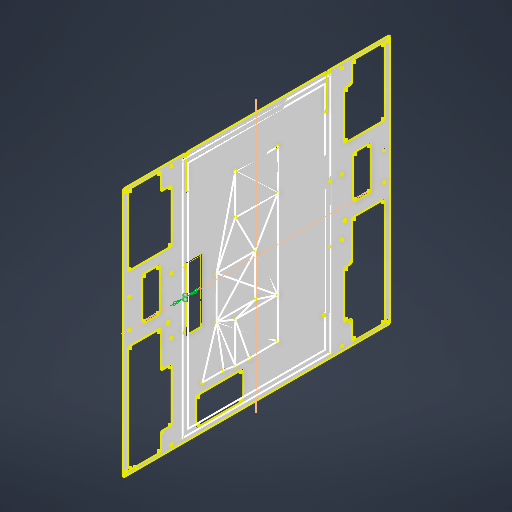
# Autodesk Inventor part: дно 25-26
Saved by Autodesk Inventor 2026.2 (Build 302298000, 298)
## iProperties
Created: 2025-09-06
Part Number: дно 25-26
Material: Типовые
Document SubType Name: Modeling
Designer: Trene
Density: 1 g/cm^3
Appearance: По умолчанию
Author: Trene
Autodesk Inventor part; units mm, degrees
(part 1 of 4)
ref_plane "YZ Plane" through (0, 0, 0) normal (1, 0, 0) x (0, 1, 0)
ref_plane "XZ Plane" through (0, 0, 0) normal (0, 1, 0) x (-1, 0, 0)
ref_plane "XY Plane" through (0, 0, 0) normal (0, 0, 1) x (1, 0, 0)
sketch "Эскиз1" plane through (0, 0, 0) normal (1, 0, 0) x (0, 1, 0)
  line L0 (0, 0) -> (370, 0)
  line L1 (370, 0) -> (370, -370)
  line L2 (370, -370) -> (0, -370)
  line L3 (0, -370) -> (0, 0)
  dimension "d0" = 370
  dimension "d1" = 370
  constraints: 8 end point, 2 parallel, 1 horizontal, 1 perpendicular
  measures "d0" distance of L1.end L2.end
  measures "d1" distance of L0.end L1.end
extrude "Выдавливание1" add sketch "Эскиз1" along normal blind 1.5
sketch "Эскиз3" plane through (1.5, 0, 0) normal (1, 0, 0) x (0, 0, -1)
  line L0 (0, 0) -> (370, 0) projected
  line L1 (8, 0) -> (50, 0)
  line L2 (50, 0) -> (50, 100)
  line L3 (50, 100) -> (8, 100)
  line L4 (8, 100) -> (8, 0)
  line L5 (0, 370) -> (0, 0) projected
  line L6 (370, 370) -> (0, 370) projected
  line L7 (185, 370) -> (185, 0)
  line L8 (0, 185) -> (370, 185)
  line L9 (370, 0) -> (370, 370) projected
  line L10 (362, 0) -> (320, 0)
  line L11 (320, 0) -> (320, 100)
  line L12 (320, 100) -> (362, 100)
  line L13 (362, 100) -> (362, 0)
  line L14 (8, 370) -> (50, 370)
  line L15 (50, 370) -> (50, 270)
  line L16 (50, 270) -> (8, 270)
  line L17 (8, 270) -> (8, 370)
  line L18 (362, 370) -> (320, 370)
  line L19 (320, 370) -> (320, 270)
  line L20 (320, 270) -> (362, 270)
  line L21 (362, 270) -> (362, 370)
  point P0 (362, 370)
  point P1 (8, 370)
  dimension "d9" = 42
  dimension "d10" = 100
  dimension "d13" = 8
  constraints: 36 end point, 12 symmetric about line, 4 midpoint, 2 parallel, 1 horizontal, 1 perpendicular, 1 point on line
  measures "d9" distance of L3.end L2.end
  measures "d10" distance of L2.end L1.end
  measures "d13" distance between parallel lines of L5 L4
extrude "Выдавливание3" cut sketch "Эскиз3" against normal blind 10 contours L4 L3 L2 L0 | L6 L15 L16 L17 | L11 L12 L13 L0 | L6 L21 L20 L19
sketch "Эскиз4" plane through (1.5, 0, 0) normal (1, 0, 0) x (0, 0, -1)
  line L0 (50, 0) -> (320, 0) projected
  line L1 (185, 0) -> (185, 257.6138)
  line L2 (0, 370) -> (0, 0) projected
  line L3 (0, 185) -> (403.9864, 185)
  line L4 (120, 370.5966) -> (250, 370.5966)
  line L5 (250, 370.5966) -> (250, 320.5966)
  line L6 (250, 320.5966) -> (120, 320.5966)
  line L7 (120, 320.5966) -> (120, 370.5966)
  line L8 (120, 370.5966) -> (250, 320.5966) construction
  line L9 (250, 370.5966) -> (120, 320.5966) construction
  point P0 (185, 370)
  point P1 (185, 305.5966)
  dimension "d62" = 50
  dimension "d63" = 130
  constraints: 12 end point, 2 midpoint, 1 horizontal, 1 symmetric about line, 1 vertical, 6 other
  measures "d62" distance between parallel lines of L4 L6
  measures "d63" distance between parallel lines of L7 L5
extrude "Выдавливание4" cut sketch "Эскиз4" against normal blind 10
sketch "Эскиз5" plane through (1.5, 0, 0) normal (1, 0, 0) x (0, 0, -1)
  line L0 (320, 370) -> (250, 370) projected
  line L1 (50, 0) -> (320, 0) projected
  line L2 (185, 0) -> (185, 405.4433)
  line L3 (50, 100) -> (50, 0) projected
  line L4 (320, 100) -> (362, 100) projected
  line L5 (320, 100) -> (362, 100)
  line L6 (362, 100) -> (362, 103)
  line L7 (362, 103) -> (320, 103)
  line L8 (320, 103) -> (320, 100)
  line L9 (50, 100) -> (8, 100)
  line L10 (50, 100) -> (8, 100)
  line L11 (8, 100) -> (8, 103)
  line L12 (8, 103) -> (50, 103)
  line L13 (50, 103) -> (50, 100)
  line L14 (0, 370) -> (0, 0) projected
  line L15 (0, 185) -> (370, 185)
  line L16 (370, 0) -> (370, 370) projected
  line L17 (50, 270) -> (50, 370)
  line L18 (320, 270) -> (362, 270)
  line L19 (320, 270) -> (362, 270)
  line L20 (362, 270) -> (362, 267)
  line L21 (362, 267) -> (320, 267)
  line L22 (320, 267) -> (320, 270)
  line L23 (50, 267) -> (50, 270)
  line L24 (8, 267) -> (50, 267)
  line L25 (50, 270) -> (8, 270)
  line L26 (50, 270) -> (8, 270)
  line L27 (8, 270) -> (8, 267)
  line L28 (320, 0) -> (320, 100) projected
  line L29 (362, 103) -> (320, 103)
  line L30 (320, 103) -> (320, 140)
  line L31 (320, 140) -> (362, 140)
  line L32 (362, 140) -> (362, 103)
  line L33 (8, 103) -> (50, 103)
  line L34 (50, 103) -> (50, 140)
  line L35 (50, 140) -> (8, 140)
  line L36 (8, 140) -> (8, 103)
  point P0 (250, 0)
  point P1 (185, -35.4433)
  dimension "d36" = 42
  dimension "d37" = 3
  constraints: 60 end point, 21 symmetric about line, 4 parallel, 3 midpoint, 2 horizontal, 2 perpendicular, 1 vertical
  measures "d36" distance of L7.end L6.end
  measures "d37" distance of L6.end L5.end
extrude "Выдавливание5" cut sketch "Эскиз5" against normal blind 10 contours L30 L31 L32 L7 | L12 L36 L35 L34
sketch "Эскиз6" plane through (1.5, 0, 0) normal (1, 0, 0) x (0, 0, -1)
  line L0 (320, 370) -> (250, 370) projected
  line L1 (299, 370) -> (259, 370)
  line L2 (259, 370) -> (259, 355)
  line L3 (259, 355) -> (299, 355)
  line L4 (299, 355) -> (299, 370)
  line L5 (250, 320.5966) -> (120, 320.5966) projected
  line L6 (185, 320.5966) -> (185, 152.8583)
  line L7 (71, 370) -> (111, 370)
  line L8 (111, 370) -> (111, 355)
  line L9 (111, 355) -> (71, 355)
  line L10 (71, 355) -> (71, 370)
  line L11 (95.25, 0) -> (95.25, 55) projected
  line L12 (95.25, 0) -> (163.25, 0)
  line L13 (163.25, 0) -> (163.25, 15)
  line L14 (163.25, 15) -> (95.25, 15)
  line L15 (95.25, 15) -> (95.25, 0)
  line L16 (8, 0) -> (50, 0)
  line L17 (50, 0) -> (50, 3)
  line L18 (50, 3) -> (8, 3)
  line L19 (8, 3) -> (8, 0)
  line L20 (362, 0) -> (320, 0)
  line L21 (320, 0) -> (320, 3)
  line L22 (320, 3) -> (362, 3)
  line L23 (362, 3) -> (362, 0)
  line L24 (370, 0) -> (370, 370) projected
  line L25 (370, 0) -> (0, 0)
  line L26 (0, 0) -> (0, -2)
  line L27 (0, -2) -> (370, -2)
  line L28 (370, -2) -> (370, 0)
  line L29 (0, 370) -> (0, 0) projected
  line L30 (0, 185) -> (370, 185)
  line L31 (370, 370) -> (0, 370)
  line L32 (0, 370) -> (0, 372)
  line L33 (0, 372) -> (370, 372)
  line L34 (370, 372) -> (370, 370)
  line L35 (50, 370) -> (50, 367)
  line L36 (50, 367) -> (8, 367)
  line L37 (8, 367) -> (8, 370)
  line L38 (320, 370) -> (320, 367)
  line L39 (320, 367) -> (362, 367)
  line L40 (362, 367) -> (362, 370)
  point P0 (362, 370)
  dimension "d28" = 40
  dimension "d29" = 15
  dimension "d32" = 68
  dimension "d33" = 15
  dimension "d34" = 42
  dimension "d35" = 3
  dimension "d38" = 370
  dimension "d39" = 2
  constraints: 72 end point, 18 symmetric about line, 8 parallel, 4 horizontal, 4 perpendicular, 3 midpoint, 1 vertical
  measures "d28" distance of L3.end L2.end
  measures "d29" distance of L2.end L1.end
  measures "d32" distance of L14.end L13.end
  measures "d33" distance of L13.end L12.end
  measures "d34" distance of L18.end L17.end
  measures "d35" distance of L17.end L16.end
  measures "d38" distance of L27.end L26.end
  measures "d39" distance of L26.end L25.end
extrude "Выдавливание6" add sketch "Эскиз6" against normal up to surface (1.5 mm away) contours L0 L31 L7 L32 L33 L34 | L31 L40 L39 L38 | L4 L3 L2 L0 | L8 L9 L10 L7 | L28 L27 L26 L25 L16 L12 L20 | L20 L21 L22 L23 | L35 L36 L37 L31 | L12 L11 L14 L13 | L19 L18 L17 L16
sketch "Эскиз7" plane through (0, 0, 0) normal (-1, 0, 0) x (0, 0, 1)
  line L0 (0, -2) -> (0, 372) projected
  line L1 (0, 372) -> (-370, 372) projected
  line L2 (-370, -2) -> (-370, 372) projected
  line L3 (-370, -2) -> (0, -2) projected
  line L4 (-362, 3) -> (-362, 100) projected
  line L5 (-320, 100) -> (-320, 3) projected
  line L6 (-320, 3) -> (-362, 3) projected
  line L7 (-320, 367) -> (-320, 270) projected
  line L8 (-362, 270) -> (-362, 367) projected
  line L9 (-362, 367) -> (-320, 367) projected
  line L10 (-250, 370) -> (-120, 370) projected
  line L11 (-120, 370) -> (-120, 320.5966) projected
  line L12 (-120, 320.5966) -> (-250, 320.5966) projected
  line L13 (-250, 320.5966) -> (-250, 370) projected
  line L14 (-8, 3) -> (-50, 3) projected
  line L15 (-50, 3) -> (-50, 100) projected
  line L16 (-8, 100) -> (-8, 3) projected
  line L17 (-50, 367) -> (-8, 367) projected
  line L18 (-8, 367) -> (-8, 270) projected
  line L19 (-50, 270) -> (-50, 367) projected
  line L20 (0, 15) -> (-370, 15)
  line L21 (-362, 100) -> (-320, 100) projected
  line L22 (-320, 270) -> (-362, 270) projected
  line L23 (-50, 100) -> (-8, 100) projected
  line L24 (-8, 270) -> (-50, 270) projected
  point P0 (0, 0)
  point P1 (-8, 15)
  point P2 (-50, 15)
  point P3 (-320, 15)
  point P4 (-362, 15)
  constraints: 2 end point, 2 point on line, 1 perpendicular
extrude "Выдавливание7" cut sketch "Эскиз7" against normal blind 10 contours L3 L2 L20 L4 L6 L5 L15 L14 L16 L0 | L20 L15 L23 L16 | L16 L14 L15 L20 | L20 L5 L6 L4
sketch "Эскиз8" plane through (1.5, 0, 0) normal (1, 0, 0) x (0, 0, -1)
  line L0 (8, 103) -> (8, 140) projected
  line L1 (8, 140) -> (50, 140) projected
  line L2 (50, 140) -> (50, 103) projected
  line L3 (50, 103) -> (8, 103) projected
  line L4 (320, 103) -> (320, 140) projected
  line L5 (320, 140) -> (362, 140) projected
  line L6 (362, 140) -> (362, 103) projected
  line L7 (362, 103) -> (320, 103) projected
  line L8 (8, 367) -> (50, 367) projected
  line L9 (50, 367) -> (50, 270) projected
  line L10 (50, 270) -> (8, 270) projected
  line L11 (8, 270) -> (8, 367) projected
  line L12 (362, 15) -> (370, 15) projected
  line L13 (370, 15) -> (370, 372) projected
  line L14 (370, 372) -> (0, 372) projected
  line L15 (0, 372) -> (0, 15) projected
  line L16 (0, 15) -> (8, 15) projected
  line L17 (8, 15) -> (8, 100) projected
  line L18 (8, 100) -> (50, 100) projected
  line L19 (50, 100) -> (50, 15) projected
  line L20 (50, 15) -> (320, 15) projected
  line L21 (320, 15) -> (320, 100) projected
  line L22 (320, 100) -> (362, 100) projected
  line L23 (362, 100) -> (362, 15) projected
  line L24 (320, 367) -> (362, 367) projected
  line L25 (362, 367) -> (362, 270) projected
  line L26 (362, 270) -> (320, 270) projected
  line L27 (320, 270) -> (320, 367) projected
  line L28 (250, 370) -> (250, 320.5966) projected
  line L29 (250, 320.5966) -> (120, 320.5966) projected
  line L30 (120, 320.5966) -> (120, 370) projected
  line L31 (120, 370) -> (250, 370) projected
  line L32 (362, 100) -> (362, 103)
  line L33 (320, 100) -> (320, 103)
  line L34 (50, 100) -> (50, 103)
  line L35 (8, 100) -> (8, 103)
  line L36 (185, 15) -> (113, 15)
  line L37 (113, 15) -> (113, 60)
  line L38 (113, 60) -> (185, 60)
  line L39 (185, 60) -> (185, 15)
  point P0 (0, 0)
  point P1 (113, 15)
  dimension "d54" = 72
  dimension "d55" = 45
  dimension "d58" = 185
  constraints: 16 end point, 5 parallel, 1 horizontal, 1 midpoint, 1 perpendicular, 1 vertical
  measures "d54" distance of L37.end L38.end
  measures "d55" distance of L36.end L37.end
  measures "d58" distance between parallel lines of L15 L39
extrude "Выдавливание8" cut sketch "Эскиз8" against normal blind 10 contours L3 L34 L18 L35 | L37 L38 L39 L20 | L33 L7 L32 L22
ref_plane "РабПлоскость1" through (1.5, 185, 0) normal (0, 1, 0) x (1, 0, 0)
sketch "Эскиз9" plane through (1.5, 0, 0) normal (1, 0, 0) x (0, 0, -1)
  line L0 (50, 140) -> (50, 15) projected
  line L1 (50, 15) -> (113, 15) projected
  line L2 (113, 15) -> (113, 60) projected
  line L3 (113, 60) -> (185, 60) projected
  line L4 (185, 60) -> (185, 15) projected
  line L5 (185, 15) -> (320, 15) projected
  line L6 (320, 15) -> (320, 140) projected
  line L7 (320, 140) -> (362, 140) projected
  line L8 (362, 140) -> (362, 15) projected
  line L9 (362, 15) -> (370, 15) projected
  line L10 (370, 15) -> (370, 372) projected
  line L11 (370, 372) -> (0, 372) projected
  line L12 (0, 372) -> (0, 15) projected
  line L13 (0, 15) -> (8, 15) projected
  line L14 (8, 15) -> (8, 140) projected
  line L15 (8, 140) -> (50, 140) projected
  line L16 (8, 367) -> (50, 367) projected
  line L17 (50, 367) -> (50, 270) projected
  line L18 (50, 270) -> (8, 270) projected
  line L19 (8, 270) -> (8, 367) projected
  line L20 (320, 367) -> (362, 367) projected
  line L21 (362, 367) -> (362, 270) projected
  line L22 (362, 270) -> (320, 270) projected
  line L23 (320, 270) -> (320, 367) projected
  line L24 (250, 370) -> (250, 320.5966) projected
  line L25 (250, 320.5966) -> (120, 320.5966) projected
  line L26 (120, 320.5966) -> (120, 370) projected
  line L27 (120, 370) -> (250, 370) projected
  line L28 (-74, 185) -> (444, 185) projected
  line L29 (8, 3) -> (50, 3)
  line L30 (50, 3) -> (50, 100)
  line L31 (50, 100) -> (8, 100)
  line L32 (8, 100) -> (8, 3)
  line L33 (320, 3) -> (362, 3)
  line L34 (362, 3) -> (362, 100)
  line L35 (362, 100) -> (320, 100)
  line L36 (320, 100) -> (320, 3)
  line L37 (370, -2) -> (0, -2)
  line L38 (370, -2) -> (370, 15)
  line L39 (0, -2) -> (0, 15)
  line L40 (185, 15) -> (113, 15)
  point P0 (0, 0)
  point P1 (50, 15)
  point P2 (8, 15)
  point P3 (362, 15)
  point P4 (320, 15)
  constraints: 24 end point, 10 symmetric about line, 1 collinear, 1 parallel, 1 vertical
extrude "Выдавливание9" add sketch "Эскиз9" against normal up to surface (1.5 mm away) contours L1 L40 L5 L36 L33 L34 L9 L38 L37 L39 L13 L32 L29 L30
sketch "Эскиз10" plane through (1.5, 0, 0) normal (1, 0, 0) x (0, 0, -1)
  point P0 (0, 0)
sketch "Эскиз11" plane through (1.5, 0, 0) normal (1, 0, 0) x (0, 0, -1)
  line L0 (370, -2) -> (370, 372) projected
  line L1 (370, 372) -> (0, 372) projected
  line L2 (0, 372) -> (0, -2) projected
  line L3 (0, -2) -> (370, -2) projected
  line L4 (113, 15) -> (113, 60) projected
  line L5 (113, 60) -> (185, 60) projected
  line L6 (185, 60) -> (185, 15) projected
  line L7 (185, 15) -> (113, 15) projected
  line L8 (362, 140) -> (362, 3) projected
  line L9 (362, 3) -> (320, 3) projected
  line L10 (320, 3) -> (320, 140) projected
  line L11 (320, 140) -> (362, 140) projected
  line L12 (50, 140) -> (50, 3) projected
  line L13 (50, 3) -> (8, 3) projected
  line L14 (8, 3) -> (8, 140) projected
  line L15 (8, 140) -> (50, 140) projected
  line L16 (8, 367) -> (50, 367) projected
  line L17 (50, 367) -> (50, 270) projected
  line L18 (50, 270) -> (8, 270) projected
  line L19 (8, 270) -> (8, 367) projected
  line L20 (320, 367) -> (362, 367) projected
  line L21 (362, 367) -> (362, 270) projected
  line L22 (362, 270) -> (320, 270) projected
  line L23 (320, 270) -> (320, 367) projected
  line L24 (250, 370) -> (250, 320.5966) projected
  line L25 (250, 320.5966) -> (120, 320.5966) projected
  line L26 (120, 320.5966) -> (120, 370) projected
  line L27 (120, 370) -> (250, 370) projected
  line L28 (320, 140) -> (362, 140)
  line L29 (362, 140) -> (362, 163)
  line L30 (362, 163) -> (320, 163)
  line L31 (320, 163) -> (320, 140)
  line L32 (8, 140) -> (8, 163)
  line L33 (8, 163) -> (50, 163)
  line L34 (50, 163) -> (50, 140)
  line L35 (120, 370) -> (250, 370)
  line L36 (250, 370) -> (250, 392)
  line L37 (250, 392) -> (120, 392)
  line L38 (120, 392) -> (120, 370)
  point P0 (0, 0)
  constraints: 22 end point, 4 parallel, 3 symmetric about line, 2 horizontal, 2 perpendicular
extrude "Выдавливание10" cut sketch "Эскиз11" against normal blind 10 contours L36 L27 L38 L1 | L1 L38 L37 L36 | L11 L31 L30 L29 | L15 L32 L33 L34
sketch "Эскиз12" plane through (1.5, 0, 0) normal (1, 0, 0) x (0, 0, -1)
  line L0 (120, 320.5966) -> (120, 372) projected
  line L1 (120, 372) -> (0, 372) projected
  line L2 (0, 372) -> (0, -2) projected
  line L3 (0, -2) -> (370, -2) projected
  line L4 (370, -2) -> (370, 372) projected
  line L5 (370, 372) -> (250, 372) projected
  line L6 (250, 372) -> (250, 320.5966) projected
  line L7 (250, 320.5966) -> (120, 320.5966) projected
  line L8 (113, 15) -> (113, 60) projected
  line L9 (113, 60) -> (185, 60) projected
  line L10 (185, 60) -> (185, 15) projected
  line L11 (185, 15) -> (113, 15) projected
  line L12 (320, 3) -> (320, 163) projected
  line L13 (320, 163) -> (362, 163) projected
  line L14 (362, 163) -> (362, 3) projected
  line L15 (362, 3) -> (320, 3) projected
  line L16 (8, 3) -> (8, 163) projected
  line L17 (8, 163) -> (50, 163) projected
  line L18 (50, 163) -> (50, 3) projected
  line L19 (50, 3) -> (8, 3) projected
  line L20 (8, 367) -> (50, 367) projected
  line L21 (50, 367) -> (50, 270) projected
  line L22 (50, 270) -> (8, 270) projected
  line L23 (8, 270) -> (8, 367) projected
  line L24 (320, 367) -> (362, 367) projected
  line L25 (362, 367) -> (362, 270) projected
  line L26 (362, 270) -> (320, 270) projected
  line L27 (320, 270) -> (320, 367) projected
  line L28 (0, -2) -> (370, -2)
  line L29 (370, -2) -> (370, -5)
  line L30 (370, -5) -> (0, -5)
  line L31 (0, -5) -> (0, -2)
  line L32 (0, 372) -> (370, 372)
  line L33 (370, 372) -> (370, 375)
  line L34 (370, 375) -> (0, 375)
  line L35 (0, 375) -> (0, 372)
  line L36 (120, 372) -> (250, 372)
  line L37 (250, 372) -> (250, 394)
  line L38 (250, 394) -> (120, 394)
  line L39 (120, 394) -> (120, 372)
  point P0 (0, 0)
  point P1 (120, 375)
  point P2 (250, 375)
  constraints: 24 end point, 6 parallel, 3 horizontal, 3 perpendicular
extrude "Выдавливание11" add sketch "Эскиз12" against normal up to surface (1.5 mm away) contours L1 L35 L34 L39 | L37 L34 L33 L5 | L3 L29 L30 L31
sketch "Эскиз13" plane through (1.5, 0, 0) normal (1, 0, 0) x (0, 0, -1)
  line L0 (120, 320.5966) -> (120, 375) projected
  line L1 (120, 375) -> (0, 375) projected
  line L2 (0, 375) -> (0, -5) projected
  line L3 (0, -5) -> (370, -5) projected
  line L4 (370, -5) -> (370, 375) projected
  line L5 (370, 375) -> (250, 375) projected
  line L6 (250, 375) -> (250, 320.5966) projected
  line L7 (250, 320.5966) -> (120, 320.5966) projected
  line L8 (113, 15) -> (113, 60) projected
  line L9 (113, 60) -> (185, 60) projected
  line L10 (185, 60) -> (185, 15) projected
  line L11 (185, 15) -> (113, 15) projected
  line L12 (320, 3) -> (320, 163) projected
  line L13 (320, 163) -> (362, 163) projected
  line L14 (362, 163) -> (362, 3) projected
  line L15 (362, 3) -> (320, 3) projected
  line L16 (8, 3) -> (8, 163) projected
  line L17 (8, 163) -> (50, 163) projected
  line L18 (50, 163) -> (50, 3) projected
  line L19 (50, 3) -> (8, 3) projected
  line L20 (8, 367) -> (50, 367) projected
  line L21 (50, 367) -> (50, 270) projected
  line L22 (50, 270) -> (8, 270) projected
  line L23 (8, 270) -> (8, 367) projected
  line L24 (320, 367) -> (362, 367) projected
  line L25 (362, 367) -> (362, 270) projected
  line L26 (362, 270) -> (320, 270) projected
  line L27 (320, 270) -> (320, 367) projected
  line L28 (320, 3) -> (362, 3)
  line L29 (362, 3) -> (362, 0)
  line L30 (362, 0) -> (320, 0)
  line L31 (320, 0) -> (320, 3)
  line L32 (8, 3) -> (50, 3)
  line L33 (50, 3) -> (50, 0)
  line L34 (50, 0) -> (8, 0)
  line L35 (8, 0) -> (8, 3)
  line L36 (8, 367) -> (50, 367)
  line L37 (50, 367) -> (50, 370)
  line L38 (50, 370) -> (8, 370)
  line L39 (8, 370) -> (8, 367)
  line L40 (320, 367) -> (362, 367)
  line L41 (362, 367) -> (362, 370)
  line L42 (362, 370) -> (320, 370)
  line L43 (320, 370) -> (320, 367)
  point P0 (0, 0)
  constraints: 32 end point, 8 parallel, 4 horizontal, 4 perpendicular, 2 point on line
extrude "Выдавливание12" cut sketch "Эскиз13" against normal blind 10 contours L15 L29 L30 L31 | L19 L33 L34 L35 | L39 L38 L37 L20 | L43 L42 L41 L24
sketch "Эскиз14" plane through (1.5, 0, 0) normal (1, 0, 0) x (0, 0, -1)
  line L0 (120, 320.5966) -> (120, 375) projected
  line L1 (120, 375) -> (0, 375) projected
  line L2 (0, 375) -> (0, -5) projected
  line L3 (0, -5) -> (370, -5) projected
  line L4 (370, -5) -> (370, 375) projected
  line L5 (370, 375) -> (250, 375) projected
  line L6 (250, 375) -> (250, 320.5966) projected
  line L7 (250, 320.5966) -> (120, 320.5966) projected
  line L8 (113, 15) -> (113, 60) projected
  line L9 (113, 60) -> (185, 60) projected
  line L10 (185, 60) -> (185, 15) projected
  line L11 (185, 15) -> (113, 15) projected
  line L12 (362, 163) -> (362, 0) projected
  line L13 (362, 0) -> (320, 0) projected
  line L14 (320, 0) -> (320, 163) projected
  line L15 (320, 163) -> (362, 163) projected
  line L16 (50, 163) -> (50, 0) projected
  line L17 (50, 0) -> (8, 0) projected
  line L18 (8, 0) -> (8, 163) projected
  line L19 (8, 163) -> (50, 163) projected
  line L20 (8, 270) -> (8, 370) projected
  line L21 (8, 370) -> (50, 370) projected
  line L22 (50, 370) -> (50, 270) projected
  line L23 (50, 270) -> (8, 270) projected
  line L24 (320, 270) -> (320, 370) projected
  line L25 (320, 370) -> (362, 370) projected
  line L26 (362, 370) -> (362, 270) projected
  line L27 (362, 270) -> (320, 270) projected
  line L28 (0, 375) -> (-10, 375)
  line L29 (-10, 375) -> (-10, -5)
  line L30 (-10, -5) -> (0, -5)
  line L31 (0, -5) -> (0, 375)
  line L32 (50, 370) -> (40, 370)
  line L33 (40, 370) -> (40, 0)
  line L34 (40, 0) -> (50, 0)
  line L35 (50, 0) -> (50, 370)
  line L36 (185, 320.5966) -> (185, -45)
  line L37 (370, 375) -> (380, 375)
  line L38 (380, 375) -> (380, -5)
  line L39 (380, -5) -> (370, -5)
  line L40 (330, 370) -> (330, 0)
  point P0 (0, 0)
  point P1 (330, 270)
  point P2 (330, 163)
  point P3 (40, 270)
  point P4 (40, 163)
  constraints: 26 end point, 5 symmetric about line, 4 parallel, 2 horizontal, 2 perpendicular, 1 midpoint, 1 point on line, 1 vertical
extrude "Выдавливание13" add sketch "Эскиз14" against normal up to surface (1.5 mm away) contours L2 L30 L29 L28 | L37 L38 L39 L4 | L40 L13 L14 L15 | L16 L17 L33 L19 | L23 L33 L21 L22 | L24 L25 L40 L27
sketch "Эскиз15" plane through (1.5, 0, 0) normal (1, 0, 0) x (0, 0, -1)
  line L0 (8, 370) -> (8, 270) projected
  line L1 (8, 370) -> (-2, 370)
  line L2 (-2, 370) -> (-2, 270)
  line L3 (-2, 270) -> (8, 270)
  line L4 (8, 270) -> (8, 370)
  line L5 (120, 320.5966) -> (120, 375) projected
  line L6 (120, 375) -> (-10, 375) projected
  line L7 (-10, 375) -> (-10, -5) projected
  line L8 (-10, -5) -> (380, -5) projected
  line L9 (380, -5) -> (380, 375) projected
  line L10 (380, 375) -> (250, 375) projected
  line L11 (250, 375) -> (250, 320.5966) projected
  line L12 (250, 320.5966) -> (120, 320.5966) projected
  line L13 (113, 15) -> (113, 60) projected
  line L14 (113, 60) -> (185, 60) projected
  line L15 (185, 60) -> (185, 15) projected
  line L16 (185, 15) -> (113, 15) projected
  line L17 (362, 163) -> (362, 0) projected
  line L18 (362, 0) -> (330, 0) projected
  line L19 (330, 0) -> (330, 163) projected
  line L20 (330, 163) -> (362, 163) projected
  line L21 (40, 163) -> (40, 0) projected
  line L22 (40, 0) -> (8, 0) projected
  line L23 (8, 0) -> (8, 163) projected
  line L24 (8, 163) -> (40, 163) projected
  line L25 (8, 270) -> (8, 370) projected
  line L26 (8, 370) -> (40, 370) projected
  line L27 (40, 370) -> (40, 270) projected
  line L28 (40, 270) -> (8, 270) projected
  line L29 (330, 370) -> (362, 370) projected
  line L30 (362, 370) -> (362, 270) projected
  line L31 (362, 270) -> (330, 270) projected
  line L32 (330, 270) -> (330, 370) projected
  line L33 (8, 163) -> (-2, 163)
  line L34 (-2, 163) -> (-2, 0)
  line L35 (-2, 0) -> (8, 0)
  line L36 (8, 0) -> (8, 163)
  line L37 (185, 320.5966) -> (185, -34)
  line L38 (362, 370) -> (372, 370)
  line L39 (372, 370) -> (372, 270)
  line L40 (372, 270) -> (362, 270)
  line L41 (362, 163) -> (372, 163)
  line L42 (372, 163) -> (372, 0)
  line L43 (372, 0) -> (362, 0)
  point P0 (0, 0)
  constraints: 30 end point, 7 symmetric about line, 4 parallel, 2 horizontal, 2 perpendicular, 1 midpoint, 1 vertical
extrude "Выдавливание14" cut sketch "Эскиз15" against normal blind 10 contours L0 L3 L2 L1 | L41 L42 L43 L17 | L23 L35 L34 L33 | L38 L39 L40 L30
sketch "Эскиз16" plane through (1.5, 0, 0) normal (1, 0, 0) x (0, 0, -1)
  line L0 (120, 320.5966) -> (120, 375) projected
  line L1 (120, 375) -> (-10, 375) projected
  line L2 (-10, 375) -> (-10, -5) projected
  line L3 (-10, -5) -> (380, -5) projected
  line L4 (380, -5) -> (380, 375) projected
  line L5 (380, 375) -> (250, 375) projected
  line L6 (250, 375) -> (250, 320.5966) projected
  line L7 (250, 320.5966) -> (120, 320.5966) projected
  line L8 (113, 15) -> (113, 60) projected
  line L9 (113, 60) -> (185, 60) projected
  line L10 (185, 60) -> (185, 15) projected
  line L11 (185, 15) -> (113, 15) projected
  line L12 (330, 163) -> (372, 163) projected
  line L13 (372, 163) -> (372, 0) projected
  line L14 (372, 0) -> (330, 0) projected
  line L15 (330, 0) -> (330, 163) projected
  line L16 (40, 0) -> (-2, 0) projected
  line L17 (-2, 0) -> (-2, 163) projected
  line L18 (-2, 163) -> (40, 163) projected
  line L19 (40, 163) -> (40, 0) projected
  line L20 (40, 270) -> (-2, 270) projected
  line L21 (-2, 270) -> (-2, 370) projected
  line L22 (-2, 370) -> (40, 370) projected
  line L23 (40, 370) -> (40, 270) projected
  line L24 (330, 370) -> (372, 370) projected
  line L25 (372, 370) -> (372, 270) projected
  line L26 (372, 270) -> (330, 270) projected
  line L27 (330, 270) -> (330, 370) projected
  line L28 (113, 60) -> (93, 60)
  line L29 (93, 60) -> (93, 15)
  line L30 (93, 15) -> (113, 15)
  line L31 (113, 15) -> (113, 60)
  point P0 (0, 0)
  dimension "d74" = 20
  constraints: 8 end point, 2 parallel, 1 horizontal, 1 perpendicular
  measures "d74" distance of L30.end L29.end
extrude "Выдавливание15" cut sketch "Эскиз16" against normal blind 10 contours L30 L29 L28 L8
sketch "Эскиз17" plane through (1.5, 0, 0) normal (1, 0, 0) x (0, 0, -1)
  line L0 (185, 60) -> (93, 60) projected
  line L1 (93, 15) -> (185, 15) projected
  line L2 (185, 60) -> (165, 60)
  line L3 (165, 60) -> (165, 15)
  line L4 (165, 15) -> (185, 15)
  line L5 (185, 15) -> (185, 60)
  line L6 (93, 60) -> (185, 60)
  line L7 (185, 60) -> (185, 47)
  line L8 (185, 47) -> (93, 47)
  line L9 (93, 47) -> (93, 60)
  point P0 (0, 0)
  point P1 (165, 47)
  dimension "d81" = 13
  constraints: 16 end point, 4 parallel, 2 horizontal, 2 perpendicular, 2 point on line
  measures "d81" distance of L8.end L0.end
extrude "Выдавливание16" add sketch "Эскиз17" against normal up to surface (1.5 mm away)
sketch "Эскиз18" plane through (1.5, 0, 0) normal (1, 0, 0) x (0, 0, -1)
  line L0 (330, 370) -> (372, 370) projected
  line L1 (372, 370) -> (372, 270) projected
  line L2 (372, 270) -> (330, 270) projected
  line L3 (330, 270) -> (330, 370) projected
  line L4 (40, 270) -> (-2, 270) projected
  line L5 (-2, 270) -> (-2, 370) projected
  line L6 (-2, 370) -> (40, 370) projected
  line L7 (40, 370) -> (40, 270) projected
  line L8 (40, 0) -> (-2, 0) projected
  line L9 (-2, 0) -> (-2, 163) projected
  line L10 (-2, 163) -> (40, 163) projected
  line L11 (40, 163) -> (40, 0) projected
  line L12 (330, 163) -> (372, 163) projected
  line L13 (372, 163) -> (372, 0) projected
  line L14 (372, 0) -> (330, 0) projected
  line L15 (330, 0) -> (330, 163) projected
  line L16 (165, 15) -> (93, 15) projected
  line L17 (93, 15) -> (93, 47) projected
  line L18 (165, 47) -> (165, 15) projected
  line L19 (120, 320.5966) -> (120, 375) projected
  line L20 (120, 375) -> (-10, 375) projected
  line L21 (-10, 375) -> (-10, -5) projected
  line L22 (-10, -5) -> (380, -5) projected
  line L23 (380, -5) -> (380, 375) projected
  line L24 (380, 375) -> (250, 375) projected
  line L25 (250, 375) -> (250, 320.5966) projected
  line L26 (250, 320.5966) -> (120, 320.5966) projected
  line L27 (165, 15) -> (93, 15) projected
  line L28 (93, 15) -> (165, 15)
  line L29 (165, 15) -> (165, 5)
  line L30 (165, 5) -> (93, 5)
  line L31 (93, 5) -> (93, 15)
  line L32 (93, 47) -> (165, 47) projected
  point P0 (0, 0)
  constraints: 8 end point, 2 parallel, 1 horizontal, 1 perpendicular
extrude "Выдавливание17" cut sketch "Эскиз18" against normal blind 10 contours L29 L30 L31 L16
sketch "Эскиз19" plane through (1.5, 0, 0) normal (1, 0, 0) x (0, 0, -1)
  line L0 (120, 320.5966) -> (120, 375) projected
  line L1 (120, 375) -> (-10, 375) projected
  line L2 (-10, 375) -> (-10, -5) projected
  line L3 (-10, -5) -> (380, -5) projected
  line L4 (380, -5) -> (380, 375) projected
  line L5 (380, 375) -> (250, 375) projected
  line L6 (250, 375) -> (250, 320.5966) projected
  line L7 (250, 320.5966) -> (120, 320.5966) projected
  line L8 (165, 47) -> (165, 5) projected
  line L9 (165, 5) -> (93, 5) projected
  line L10 (93, 5) -> (93, 47) projected
  line L11 (93, 47) -> (165, 47) projected
  line L12 (330, 163) -> (372, 163) projected
  line L13 (372, 163) -> (372, 0) projected
  line L14 (372, 0) -> (330, 0) projected
  line L15 (330, 0) -> (330, 163) projected
  line L16 (40, 0) -> (-2, 0) projected
  line L17 (-2, 0) -> (-2, 163) projected
  line L18 (-2, 163) -> (40, 163) projected
  line L19 (40, 163) -> (40, 0) projected
  line L20 (40, 270) -> (-2, 270) projected
  line L21 (-2, 270) -> (-2, 370) projected
  line L22 (-2, 370) -> (40, 370) projected
  line L23 (40, 370) -> (40, 270) projected
  line L24 (330, 370) -> (372, 370) projected
  line L25 (372, 370) -> (372, 270) projected
  line L26 (372, 270) -> (330, 270) projected
  line L27 (330, 270) -> (330, 370) projected
  line L28 (-2, 375) -> (-2, 318.424)
  line L29 (-2, 270) -> (-2, 370) projected
  line L30 (-2, 318.424) -> (43, 318.424)
  line L31 (-2, 266.848) -> (40, 266.848)
  line L32 (-2, 266.848) -> (-2, 270)
  line L33 (40, 266.848) -> (40, 270)
  line L34 (185, 320.5966) -> (185, 286)
  line L35 (372, 266.848) -> (330, 266.848)
  line L36 (372, 266.848) -> (372, 270)
  line L37 (330, 266.848) -> (330, 270)
  point P0 (0, 0)
  dimension "d82" = 56.576
  constraints: 18 end point, 4 symmetric about line, 2 point on line, 2 vertical, 1 midpoint, 1 parallel, 1 perpendicular
  measures "d82" distance of L28.start L28.end
extrude "Выдавливание18" cut sketch "Эскиз19" against normal blind 10 contours L33 L31 L32 L20 | L26 L36 L35 L37
sketch "Эскиз20" plane through (0, 0, 0) normal (-1, 0, 0) x (0, 0, 1)
  line L0 (-250, 320.5966) -> (-250, 375) projected
  line L1 (-250, 375) -> (-380, 375) projected
  line L2 (-380, 375) -> (-380, -5) projected
  line L3 (-380, -5) -> (10, -5) projected
  line L4 (10, -5) -> (10, 375) projected
  line L5 (10, 375) -> (-120, 375) projected
  line L6 (-120, 375) -> (-120, 320.5966) projected
  line L7 (-120, 320.5966) -> (-250, 320.5966) projected
  line L8 (2, 370) -> (2, 266.848) projected
  line L9 (2, 266.848) -> (-40, 266.848) projected
  line L10 (-40, 266.848) -> (-40, 370) projected
  line L11 (-40, 370) -> (2, 370) projected
  line L12 (2, 0) -> (-40, 0) projected
  line L13 (-40, 0) -> (-40, 163) projected
  line L14 (-40, 163) -> (2, 163) projected
  line L15 (2, 163) -> (2, 0) projected
  line L16 (-372, 163) -> (-330, 163) projected
  line L17 (-330, 163) -> (-330, 0) projected
  line L18 (-330, 0) -> (-372, 0) projected
  line L19 (-372, 0) -> (-372, 163) projected
  line L20 (-165, 5) -> (-165, 47) projected
  line L21 (-165, 47) -> (-93, 47) projected
  line L22 (-93, 47) -> (-93, 5) projected
  line L23 (-93, 5) -> (-165, 5) projected
  line L24 (-372, 266.848) -> (-372, 370) projected
  line L25 (-372, 370) -> (-330, 370) projected
  line L26 (-330, 370) -> (-330, 266.848) projected
  line L27 (-330, 266.848) -> (-372, 266.848) projected
  line L28 (-372, 266.848) -> (-330, 266.848) projected
  line L29 (-330, 266.848) -> (-318, 266.848)
  line L30 (-318, 266.848) -> (-318, 338.848)
  line L31 (-318, 338.848) -> (-330, 338.848)
  line L32 (-330, 338.848) -> (-330, 266.848)
  line L33 (-185, 320.5966) -> (-185, -58)
  line L34 (10, 375) -> (10, -5) projected
  line L35 (10, 185) -> (-380, 185)
  line L36 (-40, 266.848) -> (-52, 266.848)
  line L37 (-52, 266.848) -> (-52, 338.848)
  line L38 (-52, 338.848) -> (-40, 338.848)
  line L39 (-330, 103.152) -> (-318, 103.152)
  line L40 (-318, 103.152) -> (-318, 31.152)
  line L41 (-318, 31.152) -> (-330, 31.152)
  line L42 (-40, 103.152) -> (-52, 103.152)
  line L43 (-52, 103.152) -> (-52, 31.152)
  line L44 (-52, 31.152) -> (-40, 31.152)
  point P0 (0, 0)
  dimension "d85" = 12
  dimension "d86" = 72
  constraints: 30 end point, 11 symmetric about line, 3 midpoint, 2 parallel, 1 horizontal, 1 perpendicular, 1 vertical
  measures "d85" distance of L31.end L30.end
  measures "d86" distance of L30.end L29.end
extrude "Выдавливание19" cut sketch "Эскиз20" against normal blind 10 contours L36 L37 L38 L10 | L44 L43 L42 L13 | L39 L40 L41 L17 | L26 L31 L30 L29
sketch "Эскиз21" plane through (0, 0, 0) normal (-1, 0, 0) x (0, 0, 1)
  circle A0 centre (-217.25, 251.9941) radius 2.1 projected
  circle A1 centre (-217.25, 312.9941) radius 2.1 projected
  circle A2 centre (-152.75, 312.9941) radius 2.1 projected
  circle A3 centre (-152.75, 251.9941) radius 2.1 projected
  circle A4 centre (-152.75, 118.0059) radius 2.1 projected
  circle A5 centre (-152.75, 57.0059) radius 2.1 projected
  circle A6 centre (-217.25, 118.0059) radius 2.1 projected
  circle A7 centre (-217.25, 57.0059) radius 2.1 projected
  point P0 (0, 0)
extrude "Выдавливание20" cut sketch "Эскиз21" against normal through all
sketch "Эскиз22" plane through (0, 0, 0) normal (-1, 0, 0) x (0, 0, 1)
  circle A0 centre (-217.25, 312.9941) radius 2.1
  circle A1 centre (-152.75, 57.0059) radius 2.1
  circle A2 centre (-152.75, 118.0059) radius 2.1
  circle A3 centre (-152.75, 312.9941) radius 2.1
  circle A4 centre (-217.25, 251.9941) radius 2.1
  circle A5 centre (-217.25, 57.0059) radius 2.1
  circle A6 centre (-217.25, 118.0059) radius 2.1
  circle A7 centre (-152.75, 251.9941) radius 2.1
  line L0 (-330, 338.848) -> (-318, 338.848)
  line L1 (-318, 338.848) -> (-318, 266.848)
  line L2 (-318, 266.848) -> (-372, 266.848)
  line L3 (-372, 266.848) -> (-372, 370)
  line L4 (-372, 370) -> (-330, 370)
  line L5 (-330, 370) -> (-330, 338.848)
  line L6 (-165, 5) -> (-165, 47)
  line L7 (-165, 47) -> (-93, 47)
  line L8 (-93, 47) -> (-93, 5)
  line L9 (-93, 5) -> (-165, 5)
  line L10 (-250, 320.5966) -> (-250, 375)
  line L11 (-250, 375) -> (-380, 375)
  line L12 (-380, 375) -> (-380, -5)
  line L13 (-380, -5) -> (10, -5)
  line L14 (10, -5) -> (10, 375)
  line L15 (10, 375) -> (-120, 375)
  line L16 (-120, 375) -> (-120, 320.5966)
  line L17 (-120, 320.5966) -> (-250, 320.5966)
  line L18 (-318, 31.152) -> (-330, 31.152)
  line L19 (-330, 31.152) -> (-330, 0)
  line L20 (-330, 0) -> (-372, 0)
  line L21 (-372, 0) -> (-372, 163)
  line L22 (-372, 163) -> (-330, 163)
  line L23 (-330, 163) -> (-330, 103.152)
  line L24 (-330, 103.152) -> (-318, 103.152)
  line L25 (-318, 103.152) -> (-318, 31.152)
  line L26 (-52, 103.152) -> (-40, 103.152)
  line L27 (-40, 103.152) -> (-40, 163)
  line L28 (-40, 163) -> (2, 163)
  line L29 (2, 163) -> (2, 0)
  line L30 (2, 0) -> (-40, 0)
  line L31 (-40, 0) -> (-40, 31.152)
  line L32 (-40, 31.152) -> (-52, 31.152)
  line L33 (-52, 31.152) -> (-52, 103.152)
  line L34 (-52, 338.848) -> (-40, 338.848)
  line L35 (-40, 338.848) -> (-40, 370)
  line L36 (-40, 370) -> (2, 370)
  line L37 (2, 370) -> (2, 266.848)
  line L38 (2, 266.848) -> (-52, 266.848)
  line L39 (-52, 266.848) -> (-52, 338.848)
  line L40 (-86.825, 191.55) -> (-86.825, 190.7483)
  spline S0 degree 3 poles (-96.825, 225.0284) (-93.4917, 225.3395) (-90.1583, 225.3808) (-86.825, 225.1507) knots 0 0 0 0 1 1 1 1
  spline S1 degree 3 poles (-86.825, 139.1519) (-90.1583, 138.7251) (-93.4917, 138.5659) (-96.825, 138.6802) knots 0 0 0 0 1 1 1 1
  line L41 (-96.825, 225.0284) -> (-96.825, 138.6802)
  line L42 (-96.825, 138.6802) -> (-86.825, 138.6802)
  line L43 (-86.825, 138.6802) -> (-86.825, 225.1507)
  line L44 (-96.825, 181.8543) -> (-86.825, 181.9155)
  line L45 (-84.825, 134.3849) -> (-98.825, 134.3849)
  line L46 (-98.825, 134.3849) -> (-98.825, 229.3849)
  line L47 (-98.825, 229.3849) -> (-84.825, 229.3849)
  line L48 (-84.825, 229.3849) -> (-84.825, 134.3849)
  line L49 (-84.825, 134.3849) -> (-98.825, 229.3849) construction
  line L50 (-98.825, 134.3849) -> (-84.825, 229.3849) construction
  circle A8 centre (-124.375, 193.0059) radius 1.85
  circle A9 centre (-124.375, 129.0059) radius 1.85
  circle A10 centre (-124.375, 129.0059) radius 2
  circle A11 centre (-124.375, 193.0059) radius 2
  point P0 (0, 0)
  point P1 (-91.825, 181.8849)
  point P2 (-86.825, 139.1519)
  point P3 (-92.633, 138.6802)
  dimension "d91" = 14
  dimension "d92" = 95
  dimension "d95" = 4
  dimension "d96" = 4
  constraints: 20 end point, 5 midpoint, 3 perpendicular, 2 centre point, 2 coincident, 2 parallel, 1 horizontal, 1 vertical
  measures "d91" distance of L46.end L47.end
  measures "d92" distance of L45.end L46.end
  measures "d95" diameter of A10
  measures "d96" diameter of A11
extrude "Выдавливание21" cut sketch "Эскиз22" against normal blind 10 contours L40 L43 L44 L41 S0 | L43 S1 L42 L41 L44 | L43 L42 S1 | S1 L42 | L45 L46 L47 L48 | A8 | A9 | A10 | A11
sketch "Эскиз23" plane through (0, 0, 0) normal (-1, 0, 0) x (0, 0, 1)
  line L0 (-337, 187.5001) -> (-337, 218.5001) projected
  line L1 (-337, 233) -> (-337, 247.5001)
  line L2 (-372, 370) -> (-372, 266.848) projected
  line L3 (-332, 247.5001) -> (-332, 187.5001)
  line L4 (-332, 187.5001) -> (-372, 187.5001)
  line L5 (-372, 187.5001) -> (-372, 247.5001)
  line L6 (-337, 247.5001) -> (-372, 247.5001)
  line L7 (-337, 247.5001) -> (-332, 247.5001)
  line L8 (-323, 233) -> (-323, 223) projected
  line L9 (-364, 233) -> (-364, 223) projected
  line L10 (-323, 233) -> (-337, 233)
  line L11 (-332, 247.5001) -> (-323, 247.5001)
  line L12 (-323, 247.5001) -> (-323, 187.5001)
  line L13 (-323, 187.5001) -> (-372, 187.5001)
  line L14 (-323, 223) -> (-364, 223)
  line L15 (-328.5, 247.5001) -> (-328.5, 187.5001)
  line L16 (-328.5, 187.5001) -> (-358.5, 187.5001)
  line L17 (-358.5, 187.5001) -> (-358.5, 247.5001)
  line L18 (-358.5, 258.4999) -> (-328.5, 187.5001) construction
  line L19 (-328.5, 258.4999) -> (-358.5, 187.5001) construction
  line L20 (-332, 187.5001) -> (-358.5, 187.5001)
  line L21 (-358.5, 187.5001) -> (-358.5, 182.5001)
  line L22 (-358.5, 182.5001) -> (-332, 182.5001)
  line L23 (-332, 182.5001) -> (-332, 187.5001)
  line L24 (-185, -235.3635) -> (-185, 601.2713)
  line L25 (-38, 247.5001) -> (-38, 187.5001)
  line L26 (-33, 247.5001) -> (2, 247.5001)
  line L27 (-33, 247.5001) -> (-38, 247.5001)
  line L28 (-11.5, 187.5001) -> (-11.5, 247.5001)
  line L29 (-38, 187.5001) -> (-11.5, 187.5001)
  line L30 (-11.5, 187.5001) -> (-11.5, 182.5001)
  line L31 (-11.5, 182.5001) -> (-38, 182.5001)
  line L32 (-38, 182.5001) -> (-38, 187.5001)
  point P0 (0, 0)
  point P1 (-343.5, 223)
  point P2 (-332, 233)
  point P3 (-332, 223)
  dimension "d97" = 60
  dimension "d98" = 40
  dimension "d101" = 30
  dimension "d102" = 26.5
  dimension "d103" = 5
  constraints: 58 end point, 10 symmetric about line, 9 point on line, 4 parallel, 4 perpendicular, 3 midpoint, 1 collinear, 1 horizontal, 1 vertical, 2 other
  measures "d97" distance of L0.start L1.end
  measures "d98" distance of L3.end L4.end
  measures "d101" distance of L15.end L16.end
  measures "d102" distance of L22.end L21.end
  measures "d103" distance of L21.end L20.end
extrude "Выдавливание22" cut sketch "Эскиз23" against normal blind 60 contours L10 L3 L14 L17 L6 L1 | L1 L7 L3 L10 | L3 L4 L17 L14 | L23 L22 L21 L4 | L27 L26 L28 L29 L25 | L29 L30 L31 L32
sketch "Эскиз25" plane through (0, 0, 0) normal (-1, 0, 0) x (0, 0, 1)
  circle A0 centre (-299, 228) radius 1.625 projected
  circle A1 centre (-316, 228) radius 1.625 projected
  circle A2 centre (-299, 368) radius 1.625 projected
  circle A3 centre (-316, 368) radius 1.625 projected
  circle A4 centre (-299, 142) radius 1.625 projected
  circle A5 centre (-316, 142) radius 1.625 projected
  circle A6 centre (-371, 228) radius 1.625 projected
  circle A7 centre (-316, 2.0002) radius 1.625 projected
  circle A8 centre (-299, 2.0002) radius 1.625 projected
  circle A9 centre (-376, 368.9) radius 2.1
  line L0 (-380, 375) -> (-380, -5) projected
  line L1 (-250, 375) -> (-380, 375) projected
  line L2 (-458, 185) -> (88, 185) projected
  circle A10 centre (-376, 1.1) radius 2.1
  line L3 (-185, -235.3635) -> (-185, 601.2713)
  circle A11 centre (-71, 228) radius 1.625
  circle A12 centre (-54, 228) radius 1.625
  circle A13 centre (-71, 368) radius 1.625
  circle A14 centre (-54, 368) radius 1.625
  circle A15 centre (-71, 142) radius 1.625
  circle A16 centre (-54, 142) radius 1.625
  circle A17 centre (1, 228) radius 1.625
  circle A18 centre (-54, 2.0002) radius 1.625
  circle A19 centre (-71, 2.0002) radius 1.625
  circle A20 centre (6, 368.9) radius 2.1
  circle A21 centre (6, 1.1) radius 2.1
  circle A22 centre (-183.175, 193.0059) radius 1.85 projected
  circle A23 centre (-183.175, 129.0059) radius 1.85 projected
  point P0 (0, 0)
  point P1 (-185, 193.309)
  point P2 (-185, 192.7028)
  dimension "d104" = 4.2
  dimension "d105" = 4
  dimension "d106" = 6.1
  constraints: 13 centre point, 12 symmetric about line, 2 end point, 1 vertical, 14 other
  measures "d104" diameter of A9
  measures "d105" distance from line of L0 A9.centre
  measures "d106" distance from line of L1 A9.centre
extrude "Выдавливание23" cut sketch "Эскиз25" against normal blind 10 contours A0 | A1 | A2 | A3 | A4 | A5 | A6 | A7 | A8 | A9 | A10 | A23 L3 | L3 A23 | L3 A22 | A11 | A12 | A13 | A14 | A15 | A16 | A17 | A18 | A19 | A20 | A21 picked at (-183.489, 193.9651)
fillet "Сопряжение1" radius 3 52 edges at (0.75, 375, 10) (0.75, -5, 10) (0.75, -5, -380) (0.75, 375, -380) (0.75, 370, -330) (0.75, 370, -372) (0.75, 338.848, -330) (0.75, 338.848, -318) (0.75, 266.848, -318) (0.75, 266.848, -372) (0.75, 320.5966, -120) (0.75, 375, -120) (0.75, 320.5966, -250) (0.75, 375, -250) (0.75, 134.3849, -98.825) (0.75, 182.5001, -38) (0.75, 182.5001, -11.5) (0.75, 247.5001, -11.5) (0.75, 247.5001, -38) (0.75, 103.152, -52) (0.75, 103.152, -40) (0.75, 47, -93) (0.75, 47, -165) (0.75, 5, -165) (0.75, 5, -93) (0.75, 0, 2) (0.75, 31.152, -52) (0.75, 31.152, -40) (0.75, 0, -40) (0.75, 163, 2) (0.75, 163, -40) (0.75, 103.152, -318) (0.75, 103.152, -330) (0.75, 31.152, -330) (0.75, 0, -330) (0.75, 31.152, -318) (0.75, 163, -330) (0.75, 163, -372) (0.75, 0, -372) (0.75, 182.5001, -332) (0.75, 247.5001, -332) (0.75, 247.5001, -358.5) (0.75, 182.5001, -358.5) (0.75, 134.3849, -84.825) (0.75, 229.3849, -98.825) (0.75, 229.3849, -84.825) (0.75, 338.848, -40) (0.75, 338.848, -52) (0.75, 370, -40) (0.75, 266.848, -52) (0.75, 266.848, 2) (0.75, 370, 2)
sketch "Эскиз26" plane through (0, 0, 0) normal (-1, 0, 0) x (0, 0, 1)
  circle A0 centre (-287, 56.343) radius 2.1 projected
  circle A1 centre (-173.9908, 56.343) radius 2.1 projected
  circle A2 centre (-319.1128, 165.0002) radius 2.1 projected
  circle A3 centre (-50.8872, 165.0002) radius 2.1 projected
  point P0 (0, 0)
extrude "Выдавливание24" cut sketch "Эскиз26" against normal blind 10
sketch "Эскиз27" plane through (0, 0, 0) normal (-1, 0, 0) x (0, 0, 1)
  circle A0 centre (-152.75, 57.0059) radius 2.1 projected
  circle A1 centre (-135.25, 60) radius 2.1
  line L0 (-162, 47) -> (-96, 47) projected
  line L1 (-145.25, 62.0059) -> (-145.25, 52.0059) projected
  circle A2 centre (-103, 60) radius 2.1
  line L2 (-93, 44) -> (-93, 8) projected
  point P0 (0, 0)
  dimension "d112" = 4.2
  dimension "d113" = 13
  dimension "d114" = 10
  dimension "d115" = 4.2
  dimension "d116" = 13
  dimension "d117" = 10
  constraints: 2 centre point
  measures "d112" diameter of A1
  measures "d113" distance from line of A1.centre L0
  measures "d114" distance from line of A1.centre L1
  measures "d115" diameter of A2
  measures "d116" distance from line of L0 A2.centre
  measures "d117" distance from line of L2 A2.centre
extrude "Выдавливание25" cut sketch "Эскиз27" against normal blind 10 contours A1 | A2
sketch "Эскиз28" plane through (0, 0, 0) normal (-1, 0, 0) x (0, 0, 1)
  circle A0 centre (-371.0468, 185.0848) radius 1.625 projected
  point P0 (0, 0)
extrude "Выдавливание26" cut sketch "Эскиз28" against normal blind 10